Autodesk Inventor part; units mm, degrees
(part 2 of 3)
  spline S132 degree 2 poles (-143.0688, -106.7013) (-143.0981, -106.8474) (-143.2409, -106.8474) knots 0 0 0 1 1 1
  spline S133 degree 2 poles (-143.2409, -106.8474) (-143.3643, -106.8474) (-143.4162, -106.6948) knots 0 0 0 1 1 1
  line L133 (-143.4162, -106.6948) -> (-143.939, -105.1234)
  line L134 (-143.939, -105.1234) -> (-144.4617, -106.6948)
  spline S134 degree 2 poles (-144.4617, -106.6948) (-144.5136, -106.8474) (-144.6403, -106.8474) knots 0 0 0 1 1 1
  spline S135 degree 2 poles (-144.6403, -106.8474) (-144.7766, -106.8474) (-144.8123, -106.6948) knots 0 0 0 1 1 1
  line L135 (-144.8123, -106.6948) -> (-145.5104, -103.5617)
  spline S136 degree 2 poles (-145.5104, -103.5617) (-145.5136, -103.539) (-145.5136, -103.5227) knots 0 0 0 1 1 1
  spline S137 degree 2 poles (-145.5136, -103.5227) (-145.5136, -103.3474) (-145.3383, -103.3474) knots 0 0 0 1 1 1
  spline S138 degree 2 poles (-145.3383, -103.3474) (-145.1987, -103.3474) (-145.1662, -103.4838) knots 0 0 0 1 1 1
  line L136 (-145.1662, -103.4838) -> (-144.6045, -106.0195)
  line L137 (-144.6045, -106.0195) -> (-144.111, -104.5422)
  spline S139 degree 2 poles (-144.111, -104.5422) (-144.0656, -104.3994) (-143.939, -104.3994) knots 0 0 0 1 1 1
  spline S140 degree 2 poles (-143.939, -104.3994) (-143.8123, -104.3994) (-143.7636, -104.5422) knots 0 0 0 1 1 1
  line L138 (-143.7636, -104.5422) -> (-143.2734, -106.0162)
  spline S141 degree 2 poles (-140.7929, -106.8474) (-141.1565, -106.8474) (-141.6662, -106.3344) (-141.6662, -105.9708) knots 0 0 0 1 2 2 2
  line L139 (-141.6662, -105.9708) -> (-141.6662, -105.6234)
  spline S142 degree 2 poles (-141.6662, -105.6234) (-141.6662, -105.1883) (-141.3156, -104.9221) knots 0 0 0 1 1 1
  spline S143 degree 2 poles (-141.3156, -104.9221) (-141.6662, -104.6558) (-141.6662, -104.2208) knots 0 0 0 1 1 1
  spline S144 degree 2 poles (-141.6662, -104.2208) (-141.6662, -103.8604) (-141.1565, -103.3474) (-140.7929, -103.3474) knots 0 0 0 1 2 2 2
  spline S145 degree 2 poles (-140.7929, -103.3474) (-140.4292, -103.3474) (-139.9195, -103.8604) (-139.9195, -104.2208) knots 0 0 0 1 2 2 2
  spline S146 degree 2 poles (-139.9195, -104.2208) (-139.9195, -104.6558) (-140.2701, -104.9221) knots 0 0 0 1 1 1
  spline S147 degree 2 poles (-140.2701, -104.9221) (-140.0169, -105.1136) (-139.9519, -105.3929) knots 0 0 0 1 1 1
  spline S148 degree 2 poles (-139.9519, -105.3929) (-139.9195, -105.5325) (-139.9195, -105.9708) knots 0 0 0 1 1 1
  spline S149 degree 2 poles (-139.9195, -105.9708) (-139.9195, -106.3344) (-140.4292, -106.8474) (-140.7929, -106.8474) knots 0 0 0 1 2 2 2
  spline S150 degree 2 poles (-140.7929, -106.4968) (-140.5753, -106.4968) (-140.2701, -106.1916) (-140.2701, -105.9708) knots 0 0 0 1 2 2 2
  line L140 (-140.2701, -105.9708) -> (-140.2701, -105.6234)
  spline S151 degree 2 poles (-140.2701, -105.6234) (-140.2701, -105.4058) (-140.5753, -105.0974) (-140.7929, -105.0974) knots 0 0 0 1 2 2 2
  spline S152 degree 2 poles (-140.7929, -105.0974) (-141.0104, -105.0974) (-141.3156, -105.4026) (-141.3156, -105.6234) knots 0 0 0 1 2 2 2
  line L141 (-141.3156, -105.6234) -> (-141.3156, -105.9708)
  spline S153 degree 2 poles (-141.3156, -105.9708) (-141.3156, -106.1916) (-141.0104, -106.4968) (-140.7929, -106.4968) knots 0 0 0 1 2 2 2
  spline S154 degree 2 poles (-140.7929, -104.7468) (-140.5753, -104.7468) (-140.2701, -104.4448) (-140.2701, -104.224) knots 0 0 0 1 2 2 2
  spline S155 degree 2 poles (-140.2701, -104.224) (-140.2701, -104.0065) (-140.5753, -103.6981) (-140.7929, -103.6981) knots 0 0 0 1 2 2 2
  spline S156 degree 2 poles (-140.7929, -103.6981) (-141.0104, -103.6981) (-141.3156, -104.0032) (-141.3156, -104.224) knots 0 0 0 1 2 2 2
  spline S157 degree 2 poles (-141.3156, -104.224) (-141.3156, -104.4448) (-141.0104, -104.7468) (-140.7929, -104.7468) knots 0 0 0 1 2 2 2
  spline S158 degree 2 poles (-138.6922, -106.8474) (-138.7604, -106.8474) (-138.8675, -106.7403) (-138.8675, -106.6721) knots 0 0 0 1 2 2 2
  spline S159 degree 2 poles (-138.8675, -106.6721) (-138.8675, -106.5519) (-138.7799, -106.5227) knots 0 0 0 1 1 1
  spline S160 degree 2 poles (-138.7799, -106.5227) (-138.5916, -106.4578) (-138.4649, -106.3766) knots 0 0 0 1 1 1
  spline S161 degree 2 poles (-138.4649, -106.3766) (-137.9, -106.0097) (-137.8351, -105.4481) knots 0 0 0 1 1 1
  line L142 (-137.8351, -105.4481) -> (-138.3448, -105.4481)
  spline S162 degree 2 poles (-138.3448, -105.4481) (-138.7084, -105.4481) (-139.2182, -104.9351) (-139.2182, -104.5714) knots 0 0 0 1 2 2 2
  line L143 (-139.2182, -104.5714) -> (-139.2182, -104.224)
  spline S163 degree 2 poles (-139.2182, -104.224) (-139.2182, -103.8604) (-138.7084, -103.3474) (-138.3448, -103.3474) knots 0 0 0 1 2 2 2
  spline S164 degree 2 poles (-138.3448, -103.3474) (-137.9812, -103.3474) (-137.4714, -103.8539) (-137.4714, -104.2175) knots 0 0 0 1 2 2 2
  line L144 (-137.4714, -104.2175) -> (-137.4714, -105.2727)
  spline S165 degree 2 poles (-137.4714, -105.2727) (-137.4714, -106.1623) (-138.2994, -106.6818) knots 0 0 0 1 1 1
  spline S166 degree 2 poles (-138.2994, -106.6818) (-138.5656, -106.8474) (-138.6922, -106.8474) knots 0 0 0 1 1 1
  line L145 (-137.8221, -105.0974) -> (-137.8221, -104.224)
  spline S167 degree 2 poles (-137.8221, -104.224) (-137.8221, -104.0065) (-138.1273, -103.6981) (-138.3448, -103.6981) knots 0 0 0 1 2 2 2
  spline S168 degree 2 poles (-138.3448, -103.6981) (-138.5623, -103.6981) (-138.8675, -104.0065) (-138.8675, -104.224) knots 0 0 0 1 2 2 2
  line L146 (-138.8675, -104.224) -> (-138.8675, -104.5714)
  spline S169 degree 2 poles (-138.8675, -104.5714) (-138.8675, -104.7922) (-138.5623, -105.0974) (-138.3448, -105.0974) knots 0 0 0 1 2 2 2
  line L147 (-138.3448, -105.0974) -> (-137.8221, -105.0974)
  spline S170 degree 2 poles (-135.0234, -105.0974) (-135.0234, -105.724) (-135.176, -106.1786) knots 0 0 0 1 1 1
  spline S171 degree 2 poles (-135.176, -106.1786) (-135.4032, -106.8474) (-135.8968, -106.8474) knots 0 0 0 1 1 1
  spline S172 degree 2 poles (-135.8968, -106.8474) (-136.3903, -106.8474) (-136.6175, -106.1818) knots 0 0 0 1 1 1
  spline S173 degree 2 poles (-136.6175, -106.1818) (-136.7701, -105.7273) (-136.7701, -105.0974) knots 0 0 0 1 1 1
  spline S174 degree 2 poles (-136.7701, -105.0974) (-136.7701, -104.4675) (-136.6175, -104.013) knots 0 0 0 1 1 1
  spline S175 degree 2 poles (-136.6175, -104.013) (-136.3903, -103.3474) (-135.8968, -103.3474) knots 0 0 0 1 1 1
  spline S176 degree 2 poles (-135.8968, -103.3474) (-135.4032, -103.3474) (-135.176, -104.0162) knots 0 0 0 1 1 1
  spline S177 degree 2 poles (-135.176, -104.0162) (-135.0234, -104.4708) (-135.0234, -105.0974) knots 0 0 0 1 1 1
  spline S178 degree 2 poles (-135.374, -105.0974) (-135.374, -104.6623) (-135.4649, -104.2792) knots 0 0 0 1 1 1
  spline S179 degree 2 poles (-135.4649, -104.2792) (-135.6078, -103.6981) (-135.8968, -103.6981) knots 0 0 0 1 1 1
  spline S180 degree 2 poles (-135.8968, -103.6981) (-136.1857, -103.6981) (-136.3253, -104.2825) knots 0 0 0 1 1 1
  spline S181 degree 2 poles (-136.3253, -104.2825) (-136.4195, -104.6721) (-136.4195, -105.0974) knots 0 0 0 1 1 1
  spline S182 degree 2 poles (-136.4195, -105.0974) (-136.4195, -105.5292) (-136.3286, -105.9156) knots 0 0 0 1 1 1
  spline S183 degree 2 poles (-136.3286, -105.9156) (-136.1857, -106.4968) (-135.8968, -106.4968) knots 0 0 0 1 1 1
  spline S184 degree 2 poles (-135.8968, -106.4968) (-135.6078, -106.4968) (-135.4649, -105.9156) knots 0 0 0 1 1 1
  spline S185 degree 2 poles (-135.4649, -105.9156) (-135.374, -105.5292) (-135.374, -105.0974) knots 0 0 0 1 1 1
  line L148 (-132.7474, -105.974) -> (-134.1468, -105.974)
  spline S186 degree 2 poles (-134.1468, -105.974) (-134.3221, -105.974) (-134.3221, -105.7987) knots 0 0 0 1 1 1
  spline S187 degree 2 poles (-134.3221, -105.7987) (-134.3221, -105.6234) (-134.1468, -105.6234) knots 0 0 0 1 1 1
  line L149 (-134.1468, -105.6234) -> (-132.7474, -105.6234)
  spline S188 degree 2 poles (-132.7474, -105.6234) (-132.5721, -105.6234) (-132.5721, -105.7987) knots 0 0 0 1 1 1
  spline S189 degree 2 poles (-132.5721, -105.7987) (-132.5721, -105.974) (-132.7474, -105.974) knots 0 0 0 1 1 1
  spline S190 degree 2 poles (-129.426, -106.6721) (-129.426, -106.8474) (-129.6013, -106.8474) knots 0 0 0 1 1 1
  spline S191 degree 2 poles (-129.6013, -106.8474) (-129.7279, -106.8474) (-129.7669, -106.7273) knots 0 0 0 1 1 1
  line L150 (-129.7669, -106.7273) -> (-130.0201, -105.974)
  line L151 (-130.0201, -105.974) -> (-131.2799, -105.974)
  line L152 (-131.2799, -105.974) -> (-131.5331, -106.7273)
  spline S192 degree 2 poles (-131.5331, -106.7273) (-131.5721, -106.8474) (-131.6987, -106.8474) knots 0 0 0 1 1 1
  spline S193 degree 2 poles (-131.6987, -106.8474) (-131.874, -106.8474) (-131.874, -106.6721) knots 0 0 0 1 1 1
  spline S194 degree 2 poles (-131.874, -106.6721) (-131.874, -106.6396) (-131.8675, -106.6169) knots 0 0 0 1 1 1
  line L153 (-131.8675, -106.6169) -> (-130.8253, -103.487)
  spline S195 degree 2 poles (-130.8253, -103.487) (-130.7766, -103.3474) (-130.65, -103.3474) knots 0 0 0 1 1 1
  spline S196 degree 2 poles (-130.65, -103.3474) (-130.5234, -103.3474) (-130.4779, -103.4838) knots 0 0 0 1 1 1
  line L154 (-130.4779, -103.4838) -> (-129.4325, -106.6169)
  spline S197 degree 2 poles (-129.4325, -106.6169) (-129.426, -106.6396) (-129.426, -106.6721) knots 0 0 0 1 1 1
  line L155 (-130.65, -104.0812) -> (-131.163, -105.6234)
  line L156 (-131.163, -105.6234) -> (-130.137, -105.6234)
  line L157 (-130.137, -105.6234) -> (-130.65, -104.0812)
  spline S198 degree 2 poles (-126.2734, -105.0974) (-126.2734, -105.6299) (-126.1695, -106.1526) knots 0 0 0 1 1 1
  spline S199 degree 2 poles (-126.1695, -106.1526) (-126.1078, -106.4643) (-125.9357, -106.961) knots 0 0 0 1 1 1
  spline S200 degree 2 poles (-125.9357, -106.961) (-125.9227, -106.9968) (-125.9227, -107.0227) knots 0 0 0 1 1 1
  spline S201 degree 2 poles (-125.9227, -107.0227) (-125.9227, -107.0942) (-126.0299, -107.1981) (-126.1013, -107.1981) knots 0 0 0 1 2 2 2
  spline S202 degree 2 poles (-126.1013, -107.1981) (-126.2117, -107.1981) (-126.2507, -107.1169) knots 0 0 0 1 1 1
  spline S203 degree 2 poles (-126.2507, -107.1169) (-126.3968, -106.8019) (-126.624, -105.6786) (-126.624, -105.0974) knots 0 0 0 1 2 2 2
  spline S204 degree 2 poles (-126.624, -105.0974) (-126.624, -104.5195) (-126.3968, -103.3961) (-126.2507, -103.0812) knots 0 0 0 1 2 2 2
  spline S205 degree 2 poles (-126.2507, -103.0812) (-126.2117, -103) (-126.1013, -103) knots 0 0 0 1 1 1
  spline S206 degree 2 poles (-126.1013, -103) (-125.9227, -103) (-125.9227, -103.1753) knots 0 0 0 1 1 1
  spline S207 degree 2 poles (-125.9227, -103.1753) (-125.9227, -103.2013) (-125.9357, -103.237) knots 0 0 0 1 1 1
  spline S208 degree 2 poles (-125.9357, -103.237) (-126.1078, -103.7338) (-126.1695, -104.0455) knots 0 0 0 1 1 1
  spline S209 degree 2 poles (-126.1695, -104.0455) (-126.2734, -104.5682) (-126.2734, -105.0974) knots 0 0 0 1 1 1
  spline S210 degree 2 poles (-124.0007, -106.8474) (-124.1273, -106.8474) (-124.1727, -106.711) knots 0 0 0 1 1 1
  line L158 (-124.1727, -106.711) -> (-125.2182, -103.5779)
  spline S211 degree 2 poles (-125.2182, -103.5779) (-125.2247, -103.5552) (-125.2247, -103.5227) knots 0 0 0 1 1 1
  spline S212 degree 2 poles (-125.2247, -103.5227) (-125.2247, -103.3474) (-125.0494, -103.3474) knots 0 0 0 1 1 1
  spline S213 degree 2 poles (-125.0494, -103.3474) (-124.9227, -103.3474) (-124.8838, -103.4675) knots 0 0 0 1 1 1
  line L159 (-124.8838, -103.4675) -> (-124.0007, -106.1169)
  line L160 (-124.0007, -106.1169) -> (-123.1175, -103.4675)
  spline S214 degree 2 poles (-123.1175, -103.4675) (-123.0786, -103.3474) (-122.9519, -103.3474) knots 0 0 0 1 1 1
  spline S215 degree 2 poles (-122.9519, -103.3474) (-122.7766, -103.3474) (-122.7766, -103.5227) knots 0 0 0 1 1 1
  spline S216 degree 2 poles (-122.7766, -103.5227) (-122.7766, -103.5552) (-122.7831, -103.5779) knots 0 0 0 1 1 1
  line L161 (-122.7831, -103.5779) -> (-123.8286, -106.711)
  spline S217 degree 2 poles (-123.8286, -106.711) (-123.874, -106.8474) (-124.0007, -106.8474) knots 0 0 0 1 1 1
  line L162 (-121.3773, -103.9448) -> (-121.7799, -104.3474)
  spline S218 degree 2 poles (-121.7799, -104.3474) (-121.8318, -104.3961) (-121.9032, -104.3961) knots 0 0 0 1 1 1
  spline S219 degree 2 poles (-121.9032, -104.3961) (-122.0786, -104.3961) (-122.0786, -104.2208) knots 0 0 0 1 1 1
  spline S220 degree 2 poles (-122.0786, -104.2208) (-122.0786, -104.1494) (-122.0266, -104.1006) knots 0 0 0 1 1 1
  line L163 (-122.0266, -104.1006) -> (-121.3416, -103.4156)
  spline S221 degree 2 poles (-121.3416, -103.4156) (-121.2734, -103.3474) (-121.2019, -103.3474) knots 0 0 0 1 1 1
  spline S222 degree 2 poles (-121.2019, -103.3474) (-121.0266, -103.3474) (-121.0266, -103.5227) knots 0 0 0 1 1 1
  line L164 (-121.0266, -103.5227) -> (-121.0266, -106.6721)
  spline S223 degree 2 poles (-121.0266, -106.6721) (-121.0266, -106.8474) (-121.2019, -106.8474) knots 0 0 0 1 1 1
  spline S224 degree 2 poles (-121.2019, -106.8474) (-121.3773, -106.8474) (-121.3773, -106.6721) knots 0 0 0 1 1 1
  line L165 (-121.3773, -106.6721) -> (-121.3773, -103.9448)
  spline S225 degree 2 poles (-120.3253, -106.4968) (-120.3253, -106.3214) (-120.15, -106.3214) knots 0 0 0 1 1 1
  spline S226 degree 2 poles (-120.15, -106.3214) (-119.9747, -106.3214) (-119.9747, -106.4968) knots 0 0 0 1 1 1
  line L166 (-119.9747, -106.4968) -> (-119.9747, -106.6721)
  spline S227 degree 2 poles (-119.9747, -106.6721) (-119.9747, -106.8474) (-120.15, -106.8474) knots 0 0 0 1 1 1
  spline S228 degree 2 poles (-120.15, -106.8474) (-120.3253, -106.8474) (-120.3253, -106.6721) knots 0 0 0 1 1 1
  line L167 (-120.3253, -106.6721) -> (-120.3253, -106.4968)
  spline S229 degree 2 poles (-118.0558, -103.3474) (-117.8805, -103.3474) (-117.8805, -103.5227) knots 0 0 0 1 1 1
  spline S230 degree 2 poles (-117.8805, -103.5227) (-117.8805, -103.6526) (-117.9682, -103.6721) knots 0 0 0 1 1 1
  spline S231 degree 2 poles (-117.9682, -103.6721) (-118.3545, -103.7727) (-118.6468, -104.1396) knots 0 0 0 1 1 1
  spline S232 degree 2 poles (-118.6468, -104.1396) (-118.8773, -104.4318) (-118.913, -104.7468) knots 0 0 0 1 1 1
  line L168 (-118.913, -104.7468) -> (-118.4032, -104.7468)
  spline S233 degree 2 poles (-118.4032, -104.7468) (-118.0331, -104.7468) (-117.5299, -105.2565) (-117.5299, -105.6234) knots 0 0 0 1 2 2 2
  line L169 (-117.5299, -105.6234) -> (-117.5299, -105.9708)
  spline S234 degree 2 poles (-117.5299, -105.9708) (-117.5299, -106.3377) (-118.0396, -106.8474) (-118.4032, -106.8474) knots 0 0 0 1 2 2 2
  spline S235 degree 2 poles (-118.4032, -106.8474) (-118.7669, -106.8474) (-119.2766, -106.3409) (-119.2766, -105.9773) knots 0 0 0 1 2 2 2
  line L170 (-119.2766, -105.9773) -> (-119.2766, -104.9221)
  spline S236 degree 2 poles (-119.2766, -104.9221) (-119.2766, -104.3279) (-118.8838, -103.8799) knots 0 0 0 1 1 1
  spline S237 degree 2 poles (-118.8838, -103.8799) (-118.5753, -103.5325) (-118.2149, -103.3864) knots 0 0 0 1 1 1
  spline S238 degree 2 poles (-118.2149, -103.3864) (-118.111, -103.3474) (-118.0558, -103.3474) knots 0 0 0 1 1 1
  line L171 (-118.926, -105.0974) -> (-118.926, -105.9708)
  spline S239 degree 2 poles (-118.926, -105.9708) (-118.926, -106.1916) (-118.6208, -106.4968) (-118.4032, -106.4968) knots 0 0 0 1 2 2 2
  spline S240 degree 2 poles (-118.4032, -106.4968) (-118.1857, -106.4968) (-117.8805, -106.1883) (-117.8805, -105.9708) knots 0 0 0 1 2 2 2
  line L172 (-117.8805, -105.9708) -> (-117.8805, -105.6234)
  spline S241 degree 2 poles (-117.8805, -105.6234) (-117.8805, -105.4026) (-118.1857, -105.0974) (-118.4032, -105.0974) knots 0 0 0 1 2 2 2
  line L173 (-118.4032, -105.0974) -> (-118.926, -105.0974)
  spline S242 degree 2 poles (-116.4812, -105.0974) (-116.4812, -104.5682) (-116.5851, -104.0455) knots 0 0 0 1 1 1
  spline S243 degree 2 poles (-116.5851, -104.0455) (-116.6435, -103.7532) (-116.8188, -103.237) knots 0 0 0 1 1 1
  spline S244 degree 2 poles (-116.8188, -103.237) (-116.8318, -103.2078) (-116.8318, -103.1753) knots 0 0 0 1 1 1
  spline S245 degree 2 poles (-116.8318, -103.1753) (-116.8318, -103.1039) (-116.7247, -103) (-116.6532, -103) knots 0 0 0 1 2 2 2
  spline S246 degree 2 poles (-116.6532, -103) (-116.5429, -103) (-116.5039, -103.0812) knots 0 0 0 1 1 1
  spline S247 degree 2 poles (-116.5039, -103.0812) (-116.3578, -103.3961) (-116.1305, -104.5195) (-116.1305, -105.0974) knots 0 0 0 1 2 2 2
  spline S248 degree 2 poles (-116.1305, -105.0974) (-116.1305, -105.6786) (-116.3578, -106.8019) (-116.5039, -107.1169) knots 0 0 0 1 2 2 2
  spline S249 degree 2 poles (-116.5039, -107.1169) (-116.5429, -107.1981) (-116.6532, -107.1981) knots 0 0 0 1 1 1
  spline S250 degree 2 poles (-116.6532, -107.1981) (-116.7214, -107.1981) (-116.8318, -107.0909) (-116.8318, -107.0227) knots 0 0 0 1 2 2 2
  spline S251 degree 2 poles (-116.8318, -107.0227) (-116.8318, -106.9903) (-116.8188, -106.961) knots 0 0 0 1 1 1
  spline S252 degree 2 poles (-116.8188, -106.961) (-116.6435, -106.4448) (-116.5851, -106.1526) knots 0 0 0 1 1 1
  spline S253 degree 2 poles (-116.5851, -106.1526) (-116.4812, -105.6299) (-116.4812, -105.0974) knots 0 0 0 1 1 1
  spline S254 degree 2 poles (149.8738, -101.6901) (149.8738, -101.5) (150.0529, -101.5) knots 0 0 0 1 1 1
  line L174 (150.0529, -101.5) -> (150.838, -101.5)
  spline S255 degree 2 poles (150.838, -101.5) (151.1355, -101.5) (151.5405, -101.949) (151.5405, -102.2713) knots 0 0 0 1 2 2 2
  line L175 (151.5405, -102.2713) -> (151.5405, -103.7287)
  spline S256 degree 2 poles (151.5405, -103.7287) (151.5405, -104.0482) (151.13, -104.5028) (150.838, -104.5028) knots 0 0 0 1 2 2 2
  line L176 (150.838, -104.5028) -> (150.0529, -104.5028)
  spline S257 degree 2 poles (150.0529, -104.5028) (149.8738, -104.5028) (149.8738, -104.3099) knots 0 0 0 1 1 1
  line L177 (149.8738, -104.3099) -> (149.8738, -101.6901)
  line L178 (150.2292, -101.8829) -> (150.2292, -104.1198)
  line L179 (150.2292, -104.1198) -> (150.838, -104.1198)
  spline S258 degree 2 poles (150.838, -104.1198) (150.9813, -104.1198) (151.1851, -103.8912) (151.1851, -103.7287) knots 0 0 0 1 2 2 2
  line L180 (151.1851, -103.7287) -> (151.1851, -102.2713)
  spline S259 degree 2 poles (151.1851, -102.2713) (151.1851, -102.1116) (150.9813, -101.8829) (150.838, -101.8829) knots 0 0 0 1 2 2 2
  line L181 (150.838, -101.8829) -> (150.2292, -101.8829)
  line L182 (152.0143, -104.3099) -> (152.0143, -101.6901)
  spline S260 degree 2 poles (152.0143, -101.6901) (152.0143, -101.5) (152.1934, -101.5) knots 0 0 0 1 1 1
  line L183 (152.1934, -101.5) -> (153.2402, -101.5)
  spline S261 degree 2 poles (153.2402, -101.5) (153.4165, -101.5) (153.4165, -101.6901) knots 0 0 0 1 1 1
  spline S262 degree 2 poles (153.4165, -101.6901) (153.4165, -101.8829) (153.2402, -101.8829) knots 0 0 0 1 1 1
  line L184 (153.2402, -101.8829) -> (152.3697, -101.8829)
  line L185 (152.3697, -101.8829) -> (152.3697, -102.6653)
  line L186 (152.3697, -102.6653) -> (152.9785, -102.6653)
  spline S263 degree 2 poles (152.9785, -102.6653) (153.1548, -102.6653) (153.1548, -102.8554) knots 0 0 0 1 1 1
  spline S264 degree 2 poles (153.1548, -102.8554) (153.1548, -103.0482) (152.9785, -103.0482) knots 0 0 0 1 1 1
  line L187 (152.9785, -103.0482) -> (152.3697, -103.0482)
  line L188 (152.3697, -103.0482) -> (152.3697, -104.1198)
  line L189 (152.3697, -104.1198) -> (153.2402, -104.1198)
  spline S265 degree 2 poles (153.2402, -104.1198) (153.4165, -104.1198) (153.4165, -104.3099) knots 0 0 0 1 1 1
  spline S266 degree 2 poles (153.4165, -104.3099) (153.4165, -104.5028) (153.2402, -104.5028) knots 0 0 0 1 1 1
  line L190 (153.2402, -104.5028) -> (152.1934, -104.5028)
  spline S267 degree 2 poles (152.1934, -104.5028) (152.0143, -104.5028) (152.0143, -104.3099) knots 0 0 0 1 1 1
  spline S268 degree 2 poles (153.8876, -101.6928) (153.8876, -101.5028) (154.0667, -101.5028) knots 0 0 0 1 1 1
  spline S269 degree 2 poles (154.0667, -101.5028) (154.243, -101.5028) (154.243, -101.6928) knots 0 0 0 1 1 1
  line L191 (154.243, -101.6928) -> (154.243, -104.1198)
  line L192 (154.243, -104.1198) -> (155.1135, -104.1198)
  spline S270 degree 2 poles (155.1135, -104.1198) (155.2898, -104.1198) (155.2898, -104.3099) knots 0 0 0 1 1 1
  spline S271 degree 2 poles (155.2898, -104.3099) (155.2898, -104.5028) (155.1135, -104.5028) knots 0 0 0 1 1 1
  line L193 (155.1135, -104.5028) -> (154.0667, -104.5028)
  spline S272 degree 2 poles (154.0667, -104.5028) (153.8876, -104.5028) (153.8876, -104.3099) knots 0 0 0 1 1 1
  line L194 (153.8876, -104.3099) -> (153.8876, -101.6928)
  spline S273 degree 2 poles (155.7609, -101.6901) (155.7609, -101.5) (155.9399, -101.5) knots 0 0 0 1 1 1
  line L195 (155.9399, -101.5) -> (157.2485, -101.5)
  spline S274 degree 2 poles (157.2485, -101.5) (157.4275, -101.5) (157.4275, -101.6901) knots 0 0 0 1 1 1
  spline S275 degree 2 poles (157.4275, -101.6901) (157.4275, -101.8829) (157.2485, -101.8829) knots 0 0 0 1 1 1
  line L196 (157.2485, -101.8829) -> (156.7719, -101.8829)
  line L197 (156.7719, -101.8829) -> (156.7719, -104.3099)
  spline S276 degree 2 poles (156.7719, -104.3099) (156.7719, -104.5028) (156.5956, -104.5028) knots 0 0 0 1 1 1
  spline S277 degree 2 poles (156.5956, -104.5028) (156.4165, -104.5028) (156.4165, -104.3099) knots 0 0 0 1 1 1
  line L198 (156.4165, -104.3099) -> (156.4165, -101.8829)
  line L199 (156.4165, -101.8829) -> (155.9399, -101.8829)
  spline S278 degree 2 poles (155.9399, -101.8829) (155.7609, -101.8829) (155.7609, -101.6901) knots 0 0 0 1 1 1
  spline S279 degree 2 poles (159.8298, -104.3099) (159.8298, -104.5028) (159.6507, -104.5028) knots 0 0 0 1 1 1
  spline S280 degree 2 poles (159.6507, -104.5028) (159.5212, -104.5028) (159.4799, -104.3705) knots 0 0 0 1 1 1
  line L200 (159.4799, -104.3705) -> (159.3008, -103.7755)
  line L201 (159.3008, -103.7755) -> (158.4275, -103.7755)
  line L202 (158.4275, -103.7755) -> (158.2485, -104.3705)
  spline S281 degree 2 poles (158.2485, -104.3705) (158.2099, -104.5028) (158.0804, -104.5028) knots 0 0 0 1 1 1
  spline S282 degree 2 poles (158.0804, -104.5028) (157.9014, -104.5028) (157.9014, -104.3099) knots 0 0 0 1 1 1
  spline S283 degree 2 poles (157.9014, -104.3099) (157.9014, -104.2769) (157.9096, -104.2521) knots 0 0 0 1 1 1
  line L203 (157.9096, -104.2521) -> (158.6893, -101.6515)
  spline S284 degree 2 poles (158.6893, -101.6515) (158.7333, -101.5028) (158.8656, -101.5028) knots 0 0 0 1 1 1
  spline S285 degree 2 poles (158.8656, -101.5028) (158.995, -101.5028) (159.0391, -101.646) knots 0 0 0 1 1 1
  line L204 (159.0391, -101.646) -> (159.8215, -104.2521)
  spline S286 degree 2 poles (159.8215, -104.2521) (159.8298, -104.2796) (159.8298, -104.3099) knots 0 0 0 1 1 1
  line L205 (158.8656, -102.1997) -> (158.5267, -103.3926)
  line L206 (158.5267, -103.3926) -> (159.2044, -103.3926)
  line L207 (159.2044, -103.3926) -> (158.8656, -102.1997)
  spline S287 degree 2 poles (163.5818, -103.7287) (163.5818, -104.0455) (163.1713, -104.5028) (162.8793, -104.5028) knots 0 0 0 1 2 2 2
  spline S288 degree 2 poles (162.8793, -104.5028) (162.378, -104.5028) (161.9895, -104.1722) knots 0 0 0 1 1 1
  spline S289 degree 2 poles (161.9895, -104.1722) (161.9152, -104.1116) (161.9152, -104.0179) knots 0 0 0 1 1 1
  spline S290 degree 2 poles (161.9152, -104.0179) (161.9152, -103.9435) (162.0171, -103.8278) (162.0942, -103.8278) knots 0 0 0 1 2 2 2
  spline S291 degree 2 poles (162.0942, -103.8278) (162.1383, -103.8278) (162.1989, -103.8664) knots 0 0 0 1 1 1
  spline S292 degree 2 poles (162.1989, -103.8664) (162.3063, -103.938) (162.557, -104.0647) knots 0 0 0 1 1 1
  spline S293 degree 2 poles (162.557, -104.0647) (162.6975, -104.1198) (162.8793, -104.1198) knots 0 0 0 1 1 1
  spline S294 degree 2 poles (162.8793, -104.1198) (163.0226, -104.1198) (163.2264, -103.8912) (163.2264, -103.7259) knots 0 0 0 1 2 2 2
  spline S295 degree 2 poles (163.2264, -103.7259) (163.2264, -103.489) (163.0309, -103.3788) knots 0 0 0 1 1 1
  line L208 (163.0309, -103.3788) -> (162.2953, -102.9601)
  spline S296 degree 2 poles (162.2953, -102.9601) (161.9152, -102.7424) (161.9152, -102.2713) knots 0 0 0 1 1 1
  spline S297 degree 2 poles (161.9152, -102.2713) (161.9152, -101.9573) (162.3256, -101.5) (162.6176, -101.5) knots 0 0 0 1 2 2 2
  spline S298 degree 2 poles (162.6176, -101.5) (163.097, -101.5) (163.3532, -101.668) knots 0 0 0 1 1 1
  spline S299 degree 2 poles (163.3532, -101.668) (163.4523, -101.7314) (163.4523, -101.8361) knots 0 0 0 1 1 1
  spline S300 degree 2 poles (163.4523, -101.8361) (163.4523, -101.9132) (163.3477, -102.0289) (163.2733, -102.0289) knots 0 0 0 1 2 2 2
  spline S301 degree 2 poles (163.2733, -102.0289) (163.243, -102.0289) (163.1989, -102.0096) knots 0 0 0 1 1 1
  spline S302 degree 2 poles (163.1989, -102.0096) (162.9041, -101.8829) (162.6176, -101.8829) knots 0 0 0 1 1 1
  spline S303 degree 2 poles (162.6176, -101.8829) (162.4744, -101.8829) (162.2705, -102.1088) (162.2705, -102.2713) knots 0 0 0 1 2 2 2
  spline S304 degree 2 poles (162.2705, -102.2713) (162.2705, -102.5165) (162.4606, -102.624) knots 0 0 0 1 1 1
  line L209 (162.4606, -102.624) -> (163.1989, -103.0427)
  spline S305 degree 2 poles (163.1989, -103.0427) (163.5818, -103.2603) (163.5818, -103.7287) knots 0 0 0 1 1 1
  spline S306 degree 2 poles (165.7223, -103.5826) (165.7223, -103.9628) (165.2347, -104.5028) (164.8904, -104.5028) knots 0 0 0 1 2 2 2
  spline S307 degree 2 poles (164.8904, -104.5028) (164.5433, -104.5028) (164.0556, -103.9628) (164.0556, -103.5826) knots 0 0 0 1 2 2 2
  line L210 (164.0556, -103.5826) -> (164.0556, -102.4174)
  spline S308 degree 2 poles (164.0556, -102.4174) (164.0556, -102.0399) (164.5405, -101.5) (164.8904, -101.5) knots 0 0 0 1 2 2 2
  spline S309 degree 2 poles (164.8904, -101.5) (165.2375, -101.5) (165.7223, -102.0372) (165.7223, -102.4174) knots 0 0 0 1 2 2 2
  line L211 (165.7223, -102.4174) -> (165.7223, -103.5826)
  line L212 (165.3669, -103.5826) -> (165.3669, -102.4174)
  spline S310 degree 2 poles (165.3669, -102.4174) (165.3669, -102.1915) (165.0887, -101.8829) (164.8904, -101.8829) knots 0 0 0 1 2 2 2
  spline S311 degree 2 poles (164.8904, -101.8829) (164.6893, -101.8829) (164.411, -102.1915) (164.411, -102.4174) knots 0 0 0 1 2 2 2
  line L213 (164.411, -102.4174) -> (164.411, -103.5826)
  spline S312 degree 2 poles (164.411, -103.5826) (164.411, -103.8113) (164.6893, -104.1198) (164.8904, -104.1198) knots 0 0 0 1 2 2 2
  spline S313 degree 2 poles (164.8904, -104.1198) (165.0887, -104.1198) (165.3669, -103.8113) (165.3669, -103.5826) knots 0 0 0 1 2 2 2
  spline S314 degree 2 poles (166.1961, -101.6928) (166.1961, -101.5028) (166.3752, -101.5028) knots 0 0 0 1 1 1
  spline S315 degree 2 poles (166.3752, -101.5028) (166.5515, -101.5028) (166.5515, -101.6928) knots 0 0 0 1 1 1
  line L214 (166.5515, -101.6928) -> (166.5515, -104.1198)
  line L215 (166.5515, -104.1198) -> (167.422, -104.1198)
  spline S316 degree 2 poles (167.422, -104.1198) (167.5983, -104.1198) (167.5983, -104.3099) knots 0 0 0 1 1 1
  spline S317 degree 2 poles (167.5983, -104.3099) (167.5983, -104.5028) (167.422, -104.5028) knots 0 0 0 1 1 1
  line L216 (167.422, -104.5028) -> (166.3752, -104.5028)
  spline S318 degree 2 poles (166.3752, -104.5028) (166.1961, -104.5028) (166.1961, -104.3099) knots 0 0 0 1 1 1
  line L217 (166.1961, -104.3099) -> (166.1961, -101.6928)
  spline S319 degree 2 poles (168.0694, -101.6928) (168.0694, -101.5028) (168.2485, -101.5028) knots 0 0 0 1 1 1
  spline S320 degree 2 poles (168.2485, -101.5028) (168.4248, -101.5028) (168.4248, -101.6928) knots 0 0 0 1 1 1
  line L218 (168.4248, -101.6928) -> (168.4248, -104.1198)
  line L219 (168.4248, -104.1198) -> (169.2953, -104.1198)
  spline S321 degree 2 poles (169.2953, -104.1198) (169.4716, -104.1198) (169.4716, -104.3099) knots 0 0 0 1 1 1
  spline S322 degree 2 poles (169.4716, -104.3099) (169.4716, -104.5028) (169.2953, -104.5028) knots 0 0 0 1 1 1
  line L220 (169.2953, -104.5028) -> (168.2485, -104.5028)
  spline S323 degree 2 poles (168.2485, -104.5028) (168.0694, -104.5028) (168.0694, -104.3099) knots 0 0 0 1 1 1
  line L221 (168.0694, -104.3099) -> (168.0694, -101.6928)
  line L222 (171.6094, -101.6928) -> (171.6094, -103.5826)
  spline S324 degree 2 poles (171.6094, -103.5826) (171.6094, -103.9628) (171.1218, -104.5028) (170.7774, -104.5028) knots 0 0 0 1 2 2 2
  spline S325 degree 2 poles (170.7774, -104.5028) (170.4303, -104.5028) (169.9427, -103.9628) (169.9427, -103.5826) knots 0 0 0 1 2 2 2
  line L223 (169.9427, -103.5826) -> (169.9427, -101.6928)
  spline S326 degree 2 poles (169.9427, -101.6928) (169.9427, -101.5028) (170.1218, -101.5028) knots 0 0 0 1 1 1
  spline S327 degree 2 poles (170.1218, -101.5028) (170.2981, -101.5028) (170.2981, -101.6928) knots 0 0 0 1 1 1
  line L224 (170.2981, -101.6928) -> (170.2981, -103.5826)
  spline S328 degree 2 poles (170.2981, -103.5826) (170.2981, -103.8113) (170.5763, -104.1198) (170.7774, -104.1198) knots 0 0 0 1 2 2 2
  spline S329 degree 2 poles (170.7774, -104.1198) (170.9758, -104.1198) (171.254, -103.8113) (171.254, -103.5826) knots 0 0 0 1 2 2 2
  line L225 (171.254, -103.5826) -> (171.254, -101.6928)
  spline S330 degree 2 poles (171.254, -101.6928) (171.254, -101.5028) (171.4331, -101.5028) knots 0 0 0 1 1 1
  spline S331 degree 2 poles (171.4331, -101.5028) (171.6094, -101.5028) (171.6094, -101.6928) knots 0 0 0 1 1 1
  spline S332 degree 2 poles (172.0832, -101.6901) (172.0832, -101.5) (172.2623, -101.5) knots 0 0 0 1 1 1
  line L226 (172.2623, -101.5) -> (173.5708, -101.5)
  spline S333 degree 2 poles (173.5708, -101.5) (173.7499, -101.5) (173.7499, -101.6901) knots 0 0 0 1 1 1
  spline S334 degree 2 poles (173.7499, -101.6901) (173.7499, -101.8829) (173.5708, -101.8829) knots 0 0 0 1 1 1
  line L227 (173.5708, -101.8829) -> (173.0942, -101.8829)
  line L228 (173.0942, -101.8829) -> (173.0942, -104.3099)
  spline S335 degree 2 poles (173.0942, -104.3099) (173.0942, -104.5028) (172.9179, -104.5028) knots 0 0 0 1 1 1
  spline S336 degree 2 poles (172.9179, -104.5028) (172.7388, -104.5028) (172.7388, -104.3099) knots 0 0 0 1 1 1
  line L229 (172.7388, -104.3099) -> (172.7388, -101.8829)
  line L230 (172.7388, -101.8829) -> (172.2623, -101.8829)
  spline S337 degree 2 poles (172.2623, -101.8829) (172.0832, -101.8829) (172.0832, -101.6901) knots 0 0 0 1 1 1
  spline S338 degree 2 poles (174.4028, -104.5028) (174.2237, -104.5028) (174.2237, -104.3099) knots 0 0 0 1 1 1
  line L231 (174.2237, -104.3099) -> (174.2237, -101.6928)
  spline S339 degree 2 poles (174.2237, -101.6928) (174.2237, -101.5028) (174.4028, -101.5028) knots 0 0 0 1 1 1
  spline S340 degree 2 poles (174.4028, -101.5028) (174.5791, -101.5028) (174.5791, -101.6928) knots 0 0 0 1 1 1
  line L232 (174.5791, -101.6928) -> (174.5791, -104.3099)
  spline S341 degree 2 poles (174.5791, -104.3099) (174.5791, -104.5028) (174.4028, -104.5028) knots 0 0 0 1 1 1
  spline S342 degree 2 poles (176.6948, -103.5826) (176.6948, -103.9628) (176.2072, -104.5028) (175.8628, -104.5028) knots 0 0 0 1 2 2 2
  spline S343 degree 2 poles (175.8628, -104.5028) (175.5157, -104.5028) (175.0281, -103.9628) (175.0281, -103.5826) knots 0 0 0 1 2 2 2
  line L233 (175.0281, -103.5826) -> (175.0281, -102.4174)
  spline S344 degree 2 poles (175.0281, -102.4174) (175.0281, -102.0399) (175.5129, -101.5) (175.8628, -101.5) knots 0 0 0 1 2 2 2
  spline S345 degree 2 poles (175.8628, -101.5) (176.2099, -101.5) (176.6948, -102.0372) (176.6948, -102.4174) knots 0 0 0 1 2 2 2
  line L234 (176.6948, -102.4174) -> (176.6948, -103.5826)
  line L235 (176.3394, -103.5826) -> (176.3394, -102.4174)
  spline S346 degree 2 poles (176.3394, -102.4174) (176.3394, -102.1915) (176.0612, -101.8829) (175.8628, -101.8829) knots 0 0 0 1 2 2 2
  spline S347 degree 2 poles (175.8628, -101.8829) (175.6617, -101.8829) (175.3835, -102.1915) (175.3835, -102.4174) knots 0 0 0 1 2 2 2
  line L236 (175.3835, -102.4174) -> (175.3835, -103.5826)
  spline S348 degree 2 poles (175.3835, -103.5826) (175.3835, -103.8113) (175.6617, -104.1198) (175.8628, -104.1198) knots 0 0 0 1 2 2 2
  spline S349 degree 2 poles (175.8628, -104.1198) (176.0612, -104.1198) (176.3394, -103.8113) (176.3394, -103.5826) knots 0 0 0 1 2 2 2
  line L237 (178.4799, -103.7011) -> (178.4799, -101.6928)
  spline S350 degree 2 poles (178.4799, -101.6928) (178.4799, -101.5028) (178.659, -101.5028) knots 0 0 0 1 1 1
  spline S351 degree 2 poles (178.659, -101.5028) (178.8353, -101.5028) (178.8353, -101.6928) knots 0 0 0 1 1 1
  line L238 (178.8353, -101.6928) -> (178.8353, -104.3099)
  spline S352 degree 2 poles (178.8353, -104.3099) (178.8353, -104.5028) (178.659, -104.5028) knots 0 0 0 1 1 1
  spline S353 degree 2 poles (178.659, -104.5028) (178.5488, -104.5028) (178.5019, -104.4036) knots 0 0 0 1 1 1
  line L239 (178.5019, -104.4036) -> (177.524, -102.2989)
  line L240 (177.524, -102.2989) -> (177.524, -104.3099)
  spline S354 degree 2 poles (177.524, -104.3099) (177.524, -104.5028) (177.3477, -104.5028) knots 0 0 0 1 1 1
  spline S355 degree 2 poles (177.3477, -104.5028) (177.1686, -104.5028) (177.1686, -104.3099) knots 0 0 0 1 1 1
  line L241 (177.1686, -104.3099) -> (177.1686, -101.6928)
  spline S356 degree 2 poles (177.1686, -101.6928) (177.1686, -101.5028) (177.3449, -101.5028) knots 0 0 0 1 1 1
  spline S357 degree 2 poles (177.3449, -101.5028) (177.4523, -101.5028) (177.5074, -101.6129) knots 0 0 0 1 1 1
  line L242 (177.5074, -101.6129) -> (178.4799, -103.7011)
  spline S358 degree 2 poles (180.9758, -103.7287) (180.9758, -104.0455) (180.5653, -104.5028) (180.2733, -104.5028) knots 0 0 0 1 2 2 2
  spline S359 degree 2 poles (180.2733, -104.5028) (179.7719, -104.5028) (179.3835, -104.1722) knots 0 0 0 1 1 1
  spline S360 degree 2 poles (179.3835, -104.1722) (179.3091, -104.1116) (179.3091, -104.0179) knots 0 0 0 1 1 1
  spline S361 degree 2 poles (179.3091, -104.0179) (179.3091, -103.9435) (179.411, -103.8278) (179.4882, -103.8278) knots 0 0 0 1 2 2 2
  spline S362 degree 2 poles (179.4882, -103.8278) (179.5322, -103.8278) (179.5928, -103.8664) knots 0 0 0 1 1 1
  spline S363 degree 2 poles (179.5928, -103.8664) (179.7003, -103.938) (179.951, -104.0647) knots 0 0 0 1 1 1
  spline S364 degree 2 poles (179.951, -104.0647) (180.0915, -104.1198) (180.2733, -104.1198) knots 0 0 0 1 1 1
  spline S365 degree 2 poles (180.2733, -104.1198) (180.4165, -104.1198) (180.6204, -103.8912) (180.6204, -103.7259) knots 0 0 0 1 2 2 2
  spline S366 degree 2 poles (180.6204, -103.7259) (180.6204, -103.489) (180.4248, -103.3788) knots 0 0 0 1 1 1
  line L243 (180.4248, -103.3788) -> (179.6893, -102.9601)
  spline S367 degree 2 poles (179.6893, -102.9601) (179.3091, -102.7424) (179.3091, -102.2713) knots 0 0 0 1 1 1
  spline S368 degree 2 poles (179.3091, -102.2713) (179.3091, -101.9573) (179.7196, -101.5) (180.0116, -101.5) knots 0 0 0 1 2 2 2
  spline S369 degree 2 poles (180.0116, -101.5) (180.4909, -101.5) (180.7471, -101.668) knots 0 0 0 1 1 1
  spline S370 degree 2 poles (180.7471, -101.668) (180.8463, -101.7314) (180.8463, -101.8361) knots 0 0 0 1 1 1
  spline S371 degree 2 poles (180.8463, -101.8361) (180.8463, -101.9132) (180.7416, -102.0289) (180.6672, -102.0289) knots 0 0 0 1 2 2 2
  spline S372 degree 2 poles (180.6672, -102.0289) (180.6369, -102.0289) (180.5928, -102.0096) knots 0 0 0 1 1 1
  spline S373 degree 2 poles (180.5928, -102.0096) (180.2981, -101.8829) (180.0116, -101.8829) knots 0 0 0 1 1 1
  spline S374 degree 2 poles (180.0116, -101.8829) (179.8683, -101.8829) (179.6645, -102.1088) (179.6645, -102.2713) knots 0 0 0 1 2 2 2
  spline S375 degree 2 poles (179.6645, -102.2713) (179.6645, -102.5165) (179.8545, -102.624) knots 0 0 0 1 1 1
  line L244 (179.8545, -102.624) -> (180.5928, -103.0427)
  spline S376 degree 2 poles (180.5928, -103.0427) (180.9758, -103.2603) (180.9758, -103.7287) knots 0 0 0 1 1 1
  spline S377 degree 2 poles (155.5878, -108.1609) (155.4994, -108.1609) (155.4705, -108.0774) knots 0 0 0 1 1 1
  line L245 (155.4705, -108.0774) -> (154.9129, -106.5588)
  spline S378 degree 2 poles (154.9129, -106.5588) (154.9064, -106.5427) (154.9064, -106.5218) knots 0 0 0 1 1 1
  spline S379 degree 2 poles (154.9064, -106.5218) (154.9064, -106.4109) (155.027, -106.4109) knots 0 0 0 1 1 1
  spline S380 degree 2 poles (155.027, -106.4109) (155.1153, -106.4109) (155.1427, -106.4848) knots 0 0 0 1 1 1
  line L246 (155.1427, -106.4848) -> (155.5878, -107.7511)
  line L247 (155.5878, -107.7511) -> (156.0329, -106.4848)
  spline S381 degree 2 poles (156.0329, -106.4848) (156.0602, -106.4109) (156.1486, -106.4109) knots 0 0 0 1 1 1
  spline S382 degree 2 poles (156.1486, -106.4109) (156.2691, -106.4109) (156.2691, -106.5218) knots 0 0 0 1 1 1
  spline S383 degree 2 poles (156.2691, -106.5218) (156.2691, -106.5427) (156.2627, -106.5588) knots 0 0 0 1 1 1
  line L248 (156.2627, -106.5588) -> (155.7051, -108.0774)
  spline S384 degree 2 poles (155.7051, -108.0774) (155.6746, -108.1609) (155.5878, -108.1609) knots 0 0 0 1 1 1
  spline S385 degree 2 poles (156.7432, -108.1609) (156.6227, -108.1609) (156.6227, -108.0484) knots 0 0 0 1 1 1
  line L249 (156.6227, -108.0484) -> (156.6227, -106.5218)
  spline S386 degree 2 poles (156.6227, -106.5218) (156.6227, -106.4109) (156.7432, -106.4109) knots 0 0 0 1 1 1
  spline S387 degree 2 poles (156.7432, -106.4109) (156.8637, -106.4109) (156.8637, -106.5218) knots 0 0 0 1 1 1
  line L250 (156.8637, -106.5218) -> (156.8637, -108.0484)
  spline S388 degree 2 poles (156.8637, -108.0484) (156.8637, -108.1609) (156.7432, -108.1609) knots 0 0 0 1 1 1
  spline S389 degree 2 poles (157.8777, -108.1609) (157.7893, -108.1609) (157.7604, -108.0774) knots 0 0 0 1 1 1
  line L251 (157.7604, -108.0774) -> (157.2028, -106.5588)
  spline S390 degree 2 poles (157.2028, -106.5588) (157.1964, -106.5427) (157.1964, -106.5218) knots 0 0 0 1 1 1
  spline S391 degree 2 poles (157.1964, -106.5218) (157.1964, -106.4109) (157.3169, -106.4109) knots 0 0 0 1 1 1
  spline S392 degree 2 poles (157.3169, -106.4109) (157.4053, -106.4109) (157.4326, -106.4848) knots 0 0 0 1 1 1
  line L252 (157.4326, -106.4848) -> (157.8777, -107.7511)
  line L253 (157.8777, -107.7511) -> (158.3229, -106.4848)
  spline S393 degree 2 poles (158.3229, -106.4848) (158.3502, -106.4109) (158.4386, -106.4109) knots 0 0 0 1 1 1
  spline S394 degree 2 poles (158.4386, -106.4109) (158.5591, -106.4109) (158.5591, -106.5218) knots 0 0 0 1 1 1
  spline S395 degree 2 poles (158.5591, -106.5218) (158.5591, -106.5427) (158.5527, -106.5588) knots 0 0 0 1 1 1
  line L254 (158.5527, -106.5588) -> (157.995, -108.0774)
  spline S396 degree 2 poles (157.995, -108.0774) (157.9645, -108.1609) (157.8777, -108.1609) knots 0 0 0 1 1 1
  spline S397 degree 2 poles (160.2753, -108.0484) (160.2753, -108.1609) (160.1548, -108.1609) knots 0 0 0 1 1 1
  spline S398 degree 2 poles (160.1548, -108.1609) (160.0664, -108.1609) (160.0391, -108.0854) knots 0 0 0 1 1 1
  line L255 (160.0391, -108.0854) -> (159.9106, -107.7367)
  line L256 (159.9106, -107.7367) -> (159.2758, -107.7367)
  line L257 (159.2758, -107.7367) -> (159.1489, -108.0854)
  spline S399 degree 2 poles (159.1489, -108.0854) (159.1215, -108.1609) (159.0331, -108.1609) knots 0 0 0 1 1 1
  spline S400 degree 2 poles (159.0331, -108.1609) (158.9126, -108.1609) (158.9126, -108.0484) knots 0 0 0 1 1 1
  spline S401 degree 2 poles (158.9126, -108.0484) (158.9126, -108.0275) (158.9191, -108.0131) knots 0 0 0 1 1 1
  line L258 (158.9191, -108.0131) -> (159.4735, -106.5315)
  spline S402 degree 2 poles (159.4735, -106.5315) (159.5072, -106.4109) (159.594, -106.4109) knots 0 0 0 1 1 1
  spline S403 degree 2 poles (159.594, -106.4109) (159.6808, -106.4109) (159.7113, -106.4929) knots 0 0 0 1 1 1
  line L259 (159.7113, -106.4929) -> (160.2689, -108.0131)
  spline S404 degree 2 poles (160.2689, -108.0131) (160.2753, -108.0292) (160.2753, -108.0484) knots 0 0 0 1 1 1
  line L260 (159.594, -106.8175) -> (159.3465, -107.5133)
  line L261 (159.3465, -107.5133) -> (159.8415, -107.5133)
  line L262 (159.8415, -107.5133) -> (159.594, -106.8175)
  spline S405 degree 2 poles (163.1358, -108.0484) (163.1358, -108.1609) (163.0152, -108.1609) knots 0 0 0 1 1 1
  spline S406 degree 2 poles (163.0152, -108.1609) (162.9269, -108.1609) (162.8995, -108.0854) knots 0 0 0 1 1 1
  line L263 (162.8995, -108.0854) -> (162.771, -107.7367)
  line L264 (162.771, -107.7367) -> (162.1362, -107.7367)
  line L265 (162.1362, -107.7367) -> (162.0093, -108.0854)
  spline S407 degree 2 poles (162.0093, -108.0854) (161.982, -108.1609) (161.8936, -108.1609) knots 0 0 0 1 1 1
  spline S408 degree 2 poles (161.8936, -108.1609) (161.773, -108.1609) (161.773, -108.0484) knots 0 0 0 1 1 1
  spline S409 degree 2 poles (161.773, -108.0484) (161.773, -108.0275) (161.7795, -108.0131) knots 0 0 0 1 1 1
  line L266 (161.7795, -108.0131) -> (162.3339, -106.5315)
  spline S410 degree 2 poles (162.3339, -106.5315) (162.3676, -106.4109) (162.4544, -106.4109) knots 0 0 0 1 1 1
  spline S411 degree 2 poles (162.4544, -106.4109) (162.5412, -106.4109) (162.5717, -106.4929) knots 0 0 0 1 1 1
  line L267 (162.5717, -106.4929) -> (163.1293, -108.0131)
  spline S412 degree 2 poles (163.1293, -108.0131) (163.1358, -108.0292) (163.1358, -108.0484) knots 0 0 0 1 1 1
  line L268 (162.4544, -106.8175) -> (162.2069, -107.5133)
  line L269 (162.2069, -107.5133) -> (162.7019, -107.5133)
  line L270 (162.7019, -107.5133) -> (162.4544, -106.8175)
  spline S413 degree 2 poles (162.1475, -105.8405) (162.1475, -105.7312) (162.268, -105.7312) knots 0 0 0 1 1 1
  spline S414 degree 2 poles (162.268, -105.7312) (162.3082, -105.7312) (162.3307, -105.7456) knots 0 0 0 1 1 1
  line L271 (162.3307, -105.7456) -> (162.7067, -106.0028)
  spline S415 degree 2 poles (162.7067, -106.0028) (162.7613, -106.0397) (162.7613, -106.096) knots 0 0 0 1 1 1
  spline S416 degree 2 poles (162.7613, -106.096) (162.7613, -106.2084) (162.6408, -106.2084) knots 0 0 0 1 1 1
  spline S417 degree 2 poles (162.6408, -106.2084) (162.599, -106.2084) (162.5685, -106.186) knots 0 0 0 1 1 1
  line L272 (162.5685, -106.186) -> (162.2021, -105.9369)
  spline S418 degree 2 poles (162.2021, -105.9369) (162.1475, -105.8999) (162.1475, -105.8405) knots 0 0 0 1 1 1
  spline S419 degree 2 poles (164.754, -108.1609) (164.6335, -108.1609) (164.6335, -108.0484) knots 0 0 0 1 1 1
  line L273 (164.6335, -108.0484) -> (164.6335, -106.5218)
  spline S420 degree 2 poles (164.6335, -106.5218) (164.6335, -106.4109) (164.754, -106.4109) knots 0 0 0 1 1 1
  spline S421 degree 2 poles (164.754, -106.4109) (164.8745, -106.4109) (164.8745, -106.5218) knots 0 0 0 1 1 1
  line L274 (164.8745, -106.5218) -> (164.8745, -108.0484)
  spline S422 degree 2 poles (164.8745, -108.0484) (164.8745, -108.1609) (164.754, -108.1609) knots 0 0 0 1 1 1
  line L275 (166.1424, -107.6933) -> (166.1424, -106.5218)
  spline S423 degree 2 poles (166.1424, -106.5218) (166.1424, -106.4109) (166.2629, -106.4109) knots 0 0 0 1 1 1
  spline S424 degree 2 poles (166.2629, -106.4109) (166.3835, -106.4109) (166.3835, -106.5218) knots 0 0 0 1 1 1
  line L276 (166.3835, -106.5218) -> (166.3835, -108.0484)
  spline S425 degree 2 poles (166.3835, -108.0484) (166.3835, -108.1609) (166.2629, -108.1609) knots 0 0 0 1 1 1
  spline S426 degree 2 poles (166.2629, -108.1609) (166.1906, -108.1609) (166.1697, -108.1191) knots 0 0 0 1 1 1
  line L277 (166.1697, -108.1191) -> (165.4482, -106.8753)
  line L278 (165.4482, -106.8753) -> (165.4482, -108.0484)
  spline S427 degree 2 poles (165.4482, -108.0484) (165.4482, -108.1609) (165.3277, -108.1609) knots 0 0 0 1 1 1
  spline S428 degree 2 poles (165.3277, -108.1609) (165.2072, -108.1609) (165.2072, -108.0484) knots 0 0 0 1 1 1
  line L279 (165.2072, -108.0484) -> (165.2072, -106.5218)
  spline S429 degree 2 poles (165.2072, -106.5218) (165.2072, -106.4109) (165.3277, -106.4109) knots 0 0 0 1 1 1
  spline S430 degree 2 poles (165.3277, -106.4109) (165.3984, -106.4109) (165.437, -106.4736) knots 0 0 0 1 1 1
  line L280 (165.437, -106.4736) -> (166.1424, -107.6933)
  spline S431 degree 2 poles (167.9085, -107.6242) (167.9085, -107.8476) (167.563, -108.1609) (167.3203, -108.1609) knots 0 0 0 1 2 2 2
  spline S432 degree 2 poles (167.3203, -108.1609) (167.0761, -108.1609) (166.7322, -107.8476) (166.7322, -107.6242) knots 0 0 0 1 2 2 2
  line L281 (166.7322, -107.6242) -> (166.7322, -106.9444)
  spline S433 degree 2 poles (166.7322, -106.9444) (166.7322, -106.7227) (167.0761, -106.4093) (167.3203, -106.4093) knots 0 0 0 1 2 2 2
  spline S434 degree 2 poles (167.3203, -106.4093) (167.5646, -106.4093) (167.9085, -106.7211) (167.9085, -106.9444) knots 0 0 0 1 2 2 2
  line L282 (167.9085, -106.9444) -> (167.9085, -107.6242)
  line L283 (167.6674, -107.6242) -> (167.6674, -106.9444)
  spline S435 degree 2 poles (167.6674, -106.9444) (167.6674, -106.8143) (167.4666, -106.6327) (167.3203, -106.6327) knots 0 0 0 1 2 2 2
  spline S436 degree 2 poles (167.3203, -106.6327) (167.1741, -106.6327) (166.9732, -106.8143) (166.9732, -106.9444) knots 0 0 0 1 2 2 2
  line L284 (166.9732, -106.9444) -> (166.9732, -107.6242)
  spline S437 degree 2 poles (166.9732, -107.6242) (166.9732, -107.756) (167.1741, -107.9376) (167.3203, -107.9376) knots 0 0 0 1 2 2 2
  spline S438 degree 2 poles (167.3203, -107.9376) (167.4666, -107.9376) (167.6674, -107.756) (167.6674, -107.6242) knots 0 0 0 1 2 2 2
  spline S439 degree 2 poles (168.9386, -108.1609) (168.8502, -108.1609) (168.8213, -108.0774) knots 0 0 0 1 1 1
  line L285 (168.8213, -108.0774) -> (168.2636, -106.5588)
  spline S440 degree 2 poles (168.2636, -106.5588) (168.2572, -106.5427) (168.2572, -106.5218) knots 0 0 0 1 1 1
  spline S441 degree 2 poles (168.2572, -106.5218) (168.2572, -106.4109) (168.3777, -106.4109) knots 0 0 0 1 1 1
  spline S442 degree 2 poles (168.3777, -106.4109) (168.4661, -106.4109) (168.4934, -106.4848) knots 0 0 0 1 1 1
  line L286 (168.4934, -106.4848) -> (168.9386, -107.7511)
  line L287 (168.9386, -107.7511) -> (169.3837, -106.4848)
  spline S443 degree 2 poles (169.3837, -106.4848) (169.411, -106.4109) (169.4994, -106.4109) knots 0 0 0 1 1 1
  spline S444 degree 2 poles (169.4994, -106.4109) (169.6199, -106.4109) (169.6199, -106.5218) knots 0 0 0 1 1 1
  spline S445 degree 2 poles (169.6199, -106.5218) (169.6199, -106.5427) (169.6135, -106.5588) knots 0 0 0 1 1 1
  line L288 (169.6135, -106.5588) -> (169.0559, -108.0774)
  spline S446 degree 2 poles (169.0559, -108.0774) (169.0253, -108.1609) (168.9386, -108.1609) knots 0 0 0 1 1 1
  spline S447 degree 2 poles (171.3362, -108.0484) (171.3362, -108.1609) (171.2157, -108.1609) knots 0 0 0 1 1 1
  spline S448 degree 2 poles (171.2157, -108.1609) (171.1273, -108.1609) (171.1, -108.0854) knots 0 0 0 1 1 1
  line L289 (171.1, -108.0854) -> (170.9714, -107.7367)
  line L290 (170.9714, -107.7367) -> (170.3366, -107.7367)
  line L291 (170.3366, -107.7367) -> (170.2097, -108.0854)
  spline S449 degree 2 poles (170.2097, -108.0854) (170.1824, -108.1609) (170.094, -108.1609) knots 0 0 0 1 1 1
  spline S450 degree 2 poles (170.094, -108.1609) (169.9735, -108.1609) (169.9735, -108.0484) knots 0 0 0 1 1 1
  spline S451 degree 2 poles (169.9735, -108.0484) (169.9735, -108.0275) (169.9799, -108.0131) knots 0 0 0 1 1 1
  line L292 (169.9799, -108.0131) -> (170.5343, -106.5315)
  spline S452 degree 2 poles (170.5343, -106.5315) (170.568, -106.4109) (170.6548, -106.4109) knots 0 0 0 1 1 1
  spline S453 degree 2 poles (170.6548, -106.4109) (170.7416, -106.4109) (170.7721, -106.4929) knots 0 0 0 1 1 1
  line L293 (170.7721, -106.4929) -> (171.3298, -108.0131)
  spline S454 degree 2 poles (171.3298, -108.0131) (171.3362, -108.0292) (171.3362, -108.0484) knots 0 0 0 1 1 1
  line L294 (170.6548, -106.8175) -> (170.4073, -107.5133)
  line L295 (170.4073, -107.5133) -> (170.9023, -107.5133)
  line L296 (170.9023, -107.5133) -> (170.6548, -106.8175)
  spline S455 degree 2 poles (172.0899, -108.5) (171.9693, -108.5) (171.9693, -108.3875) knots 0 0 0 1 1 1
  spline S456 degree 2 poles (171.9693, -108.3875) (171.9693, -108.3747) (172.04, -108.14) knots 0 0 0 1 1 1
  spline S457 degree 2 poles (172.04, -108.14) (171.8986, -108.1095) (171.6897, -107.8636) (171.6897, -107.7078) knots 0 0 0 1 2 2 2
  line L297 (171.6897, -107.7078) -> (171.6897, -106.8593)
  spline S458 degree 2 poles (171.6897, -106.8593) (171.6897, -106.6729) (171.979, -106.4093) (172.1831, -106.4093) knots 0 0 0 1 2 2 2
  line L298 (172.1831, -106.4093) -> (172.5575, -106.4093)
  spline S459 degree 2 poles (172.5575, -106.4093) (172.678, -106.4093) (172.678, -106.5202) knots 0 0 0 1 1 1
  spline S460 degree 2 poles (172.678, -106.5202) (172.678, -106.6327) (172.5575, -106.6327) knots 0 0 0 1 1 1
  line L299 (172.5575, -106.6327) -> (172.1831, -106.6327)
  spline S461 degree 2 poles (172.1831, -106.6327) (172.0368, -106.6327) (171.9645, -106.7468) knots 0 0 0 1 1 1
  spline S462 degree 2 poles (171.9645, -106.7468) (171.9308, -106.7982) (171.9308, -106.8593) knots 0 0 0 1 1 1
  line L300 (171.9308, -106.8593) -> (171.9308, -107.7094)
  spline S463 degree 2 poles (171.9308, -107.7094) (171.9308, -107.8026) (172.0786, -107.9376) (172.1831, -107.9376) knots 0 0 0 1 2 2 2
  line L301 (172.1831, -107.9376) -> (172.5575, -107.9376)
  spline S464 degree 2 poles (172.5575, -107.9376) (172.678, -107.9376) (172.678, -108.0484) knots 0 0 0 1 1 1
  spline S465 degree 2 poles (172.678, -108.0484) (172.678, -108.1609) (172.5575, -108.1609) knots 0 0 0 1 1 1
  line L302 (172.5575, -108.1609) -> (172.2779, -108.1609)
  line L303 (172.2779, -108.1609) -> (172.2072, -108.4164)